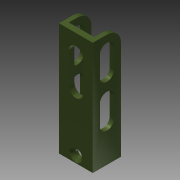
# Autodesk Inventor part: 13_1087_002
Saved by Autodesk Inventor 2014 (Build 180170000, 170)
## iProperties
Created: 2013-08-01
Part Number: 13_1087_002
Material: Kupfer
Document SubType Name: Modeling
Designer: vogel
Density: 8.94 g/cm^3
Appearance: Dunkelolivgrün
Author: vogel
Autodesk Inventor part; units mm, degrees
ref_plane "YZ Plane" through (0, 0, 0) normal (1, 0, 0) x (0, 1, 0)
ref_plane "XZ Plane" through (0, 0, 0) normal (0, 1, 0) x (-1, 0, 0)
ref_plane "XY Plane" through (0, 0, 0) normal (0, 0, 1) x (1, 0, 0)
sketch "Skizze1" plane through (0, 0, 0) normal (0, 0, 1) x (1, 0, 0)
  line L0 (-8.4, 0) -> (8.4, 0) projected
  line L1 (0, -2) -> (0, 12) projected
  line L2 (6, 10) -> (6, 0)
  line L3 (6, 0) -> (-6, 0)
  line L4 (-6, 0) -> (-6, 10)
  line L5 (4.5, 10) -> (4.5, 2)
  line L6 (4.5, 2) -> (-4.5, 2)
  line L7 (-4.5, 2) -> (-4.5, 10)
  line L8 (-6, 10) -> (-4.5, 10)
  line L9 (4.5, 10) -> (6, 10)
  point P0 (0, 0)
  dimension "d0" = 2
  dimension "d2" = 9
  dimension "d3" = 1.5
  dimension "d4" = 10
  constraints: 16 end point, 4 parallel, 2 horizontal, 2 perpendicular, 1 collinear, 1 point on line, 2 other
  measures "d0" distance between parallel lines of L0 L6
  measures "d2" distance of L5.end L6.end
  measures "d3" distance between parallel lines of L4 L7
  measures "d4" distance between parallel lines of L8 L0
extrude "Extrusion1" add sketch "Skizze1" along normal blind 40
sketch "Skizze2" plane through (-6, 0, 0) normal (0, -1, 0) x (1, 0, 0)
  line L0 (0, 0) -> (12, 0) projected
  line L1 (12, 0) -> (12, 40) projected
  point P0 (6, 0)
  point P1 (6, 2.5)
  dimension "d7" = 2.5
  dimension "d8" = 6
  measures "d7" distance from line of point (6, 2.5) L0
  measures "d8" distance from line of L1 point (6, 2.5)
hole "Bohrung1" at (0, 0, 2.5) direction (0, 1, 0) diameter 2.4 end through all countersink diameter 4.5 countersink angle 90
sketch "Skizze3" plane through (-6, 0, 0) normal (0, -1, 0) x (1, 0, 0)
  line L0 (0, 40) -> (12, 40) projected
  line L1 (0, 0) -> (0, 40) projected
  line L2 (3.5, 33.5) -> (3.5, 22.5)
  line L3 (8.5, 22.5) -> (8.5, 33.5)
  arc A0 (8.5, 33.5) -> (3.5, 33.5) centre (6, 33.5) ccw
  arc A1 (3.5, 22.5) -> (8.5, 22.5) centre (6, 22.5) ccw
  line L4 (0, 0) -> (12, 0) projected
  line L5 (6, 22.5) -> (6, 33.5)
  point P0 (6, 0)
  point P1 (6, 28)
  dimension "d36" = 4
  dimension "d37" = 20
  dimension "d38" = 6
  dimension "d39" = 5
  constraints: 6 end point, 4 point on circle, 4 tangent, 2 centre point, 1 midpoint, 1 parallel, 1 perpendicular
  measures "d36" distance edge to line of A0 L0
  measures "d38" distance from line of L1 point (6, 28)
  measures "d39" distance between parallel lines of L3 L2
extrude "Extrusion2" cut sketch "Skizze3" against normal through all
sketch "Skizze4" plane through (6, 0, 0) normal (1, 0, 0) x (0, 0, -1)
  line L0 (0, 10) -> (-40, 10) projected
  line L1 (-40, 0) -> (-40, 10) projected
  line L2 (0, 0) -> (-40, 0) projected
  line L3 (-35, 5) -> (-28, 5) construction
  line L4 (-35, 7.5) -> (-28, 7.5)
  line L5 (-28, 2.5) -> (-35, 2.5)
  arc A0 (-35, 7.5) -> (-35, 2.5) centre (-35, 5) ccw
  arc A1 (-28, 2.5) -> (-28, 7.5) centre (-28, 5) ccw
  circle A2 centre (-35, 5) radius 5
  point P0 (-31.5, 5)
  dimension "d25" = 5
  dimension "d26" = 7
  dimension "d27" = 5
  dimension "d28" = 5
  dimension "d35" = 7
  constraints: 8 end point, 5 tangent, 4 point on circle, 3 centre point, 2 parallel, 1 coincident, 1 midpoint
  measures "d25" distance from line of L1 L3.start
  measures "d26" distance of L3.start L3.end
  measures "d27" distance between parallel lines of L3 L2
  measures "d28" distance between parallel lines of L5 L4
  measures "d35" distance of L4.start L4.end
extrude "Extrusion3" cut sketch "Skizze4" against normal through all contours A2 L5 A0 L4 | L4 A1 L5 A2 picked at (-33.3333, 5)
pattern_linear "Rechteckige Anordnung1" count 2 spacing 15 along (0, 0, -1) of "Extrusion3"
fillet "Rundung1" radius 5 2 edges at (-5.25, 10, 40) (5.25, 10, 40)
